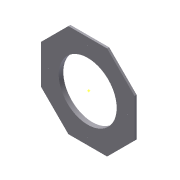
# Autodesk Inventor part: Stage3
Saved by Autodesk Inventor 2018.2 (Build 222227000, 227)
## iProperties
Created: 2018-10-31
Part Number: Stage3
Material: 3.3547 AlMg4,5Mn (AW-5083/H111)
Document SubType Name: Modeling
Designer: N.Grubert
Density: 2.66 g/cm^3
Appearance: Aluminum (gleichmäßig)
Fläche: 0 cm²
Gewicht: 0 g
Material: geeigneten Werkstoff auswählen !
Dateiname: P:\INVENTOR\Inventor 2018\Templates\ILT\Norm.ipt
Bez_eng: bolt
Bez_french: boulon
Author: N.Grubert
Autodesk Inventor part; units mm, degrees
ref_plane "YZ Plane" through (0, 0, 0) normal (1, 0, 0) x (0, 1, 0)
ref_plane "XZ Plane" through (0, 0, 0) normal (0, 1, 0) x (-1, 0, 0)
ref_plane "XY Plane" through (0, 0, 0) normal (0, 0, 1) x (1, 0, 0)
sketch "Skizze4" plane through (0, 0, 0) normal (0, 1, 0) x (-1, 0, 0)
  line L0 (-23.4031, 56.5) -> (23.4031, 56.5)
  line L1 (23.4031, 56.5) -> (56.5, 23.4031)
  line L2 (56.5, 23.4031) -> (56.5, -23.4031)
  line L3 (56.5, -23.4031) -> (23.4031, -56.5)
  line L4 (23.4031, -56.5) -> (-23.4031, -56.5)
  line L5 (-23.4031, -56.5) -> (-56.5, -23.4031)
  line L6 (-56.5, -23.4031) -> (-56.5, 23.4031)
  line L7 (-56.5, 23.4031) -> (-23.4031, 56.5)
  line L8 (0, -79.1) -> (0, 79.1) construction
  line L9 (79.1, 0) -> (-79.1, 0) construction
  circle A0 centre (0, 0) radius 35
  dimension "d4" = 113
  dimension "d5" = 70
  constraints: 16 end point, 2 coincident, 1 centre point, 18 other
  measures "d4" distance between parallel lines of L4 L0
  measures "d5" diameter of A0
extrude "Extrusion2" add sketch "Skizze4" along normal blind 2.5
sketch "Skizze5" plane through (0, 2.5, 0) normal (0, 1, 0) x (1, 0, 0)
  circle A0 centre (0, 0) radius 35 projected
  line L0 (-23.4031, -56.5) -> (23.4031, -56.5) projected
  line L1 (23.4031, -56.5) -> (56.5, -23.4031) projected
  line L2 (56.5, -23.4031) -> (56.5, 23.4031) projected
  line L3 (56.5, 23.4031) -> (23.4031, 56.5) projected
  line L4 (23.4031, 56.5) -> (-23.4031, 56.5) projected
  line L5 (-23.4031, 56.5) -> (-56.5, 23.4031) projected
  line L6 (-56.5, 23.4031) -> (-56.5, -23.4031) projected
  line L7 (-56.5, -23.4031) -> (-23.4031, -56.5) projected
  line L8 (-51.5, 21.332) -> (-21.332, 51.5)
  line L9 (-21.332, 51.5) -> (21.332, 51.5)
  line L10 (21.332, 51.5) -> (51.5, 21.332)
  line L11 (51.5, 21.332) -> (51.5, -21.332)
  line L12 (51.5, -21.332) -> (21.332, -51.5)
  line L13 (21.332, -51.5) -> (-21.332, -51.5)
  line L14 (-21.332, -51.5) -> (-51.5, -21.332)
  line L15 (-51.5, -21.332) -> (-51.5, 21.332)
  dimension "d8" = 5
  constraints: 16 end point, 7 other
  measures "d8" distance between parallel lines of L8 L5
extrude "Extrusion3" add sketch "Skizze5" along normal blind 2.5 contours L8 L9 L10 L11 L12 L13 L14 L15
sketch "Skizze6" plane through (0, 5, 0) normal (0, 1, 0) x (1, 0, 0)
  circle A0 centre (0, 0) radius 35 construction
  line L0 (-21.332, 51.5) -> (-51.5, 21.332) construction
  line L1 (-51.5, 21.332) -> (-51.5, -21.332) construction
  line L2 (-51.5, -21.332) -> (-21.332, -51.5) construction
  line L3 (-21.332, -51.5) -> (21.332, -51.5) construction
  line L4 (21.332, -51.5) -> (51.5, -21.332) construction
  line L5 (51.5, -21.332) -> (51.5, 21.332) construction
  line L6 (51.5, 21.332) -> (21.332, 51.5) construction
  line L7 (21.332, 51.5) -> (-21.332, 51.5) construction
  line L8 (0, 79.1) -> (0, -79.1) construction
  point P0 (0, 48)
  point P1 (-48, 0)
  point P2 (0, -48)
  point P3 (48, 0)
  dimension "d11" = 48
  dimension "d14" = 360
  constraints: 1 point on line, 5 other
  measures "d11" distance of point (0, 48) point (0, 0)
hole "Bohrung1" at (0, 5, -48) at (-48, 5, 0) at (0, 5, 48) at (48, 5, 0) direction (0, -1, 0) diameter 1 end through all
sketch "Skizze7" plane through (0, 2.5, 0) normal (0, 1, 0) x (1, 0, 0)
  line L0 (-21.332, 51.5) -> (21.332, 51.5) projected
  line L1 (21.332, 51.5) -> (51.5, 21.332) projected
  line L2 (51.5, 21.332) -> (51.5, -21.332) projected
  line L3 (51.5, -21.332) -> (21.332, -51.5) projected
  line L4 (21.332, -51.5) -> (-21.332, -51.5) projected
  line L5 (-21.332, -51.5) -> (-51.5, -21.332) projected
  line L6 (-51.5, -21.332) -> (-51.5, 21.332) projected
  line L7 (-51.5, 21.332) -> (-21.332, 51.5) projected
  line L8 (-23.4031, -56.5) -> (23.4031, -56.5) projected
  line L9 (23.4031, -56.5) -> (56.5, -23.4031) projected
  line L10 (56.5, -23.4031) -> (56.5, 23.4031) projected
  line L11 (56.5, 23.4031) -> (23.4031, 56.5) projected
  line L12 (23.4031, 56.5) -> (-23.4031, 56.5) projected
  line L13 (-23.4031, 56.5) -> (-56.5, 23.4031) projected
  line L14 (-56.5, 23.4031) -> (-56.5, -23.4031) projected
  line L15 (-56.5, -23.4031) -> (-23.4031, -56.5) projected
  point P0 (0, 0)
extrude "Extrusion4" cut sketch "Skizze7" against normal blind 1
sketch "Skizze8" plane through (0, 0, 0) normal (0, -1, 0) x (1, 0, 0)
  circle A0 centre (0, 48) radius 0.5 projected
  circle A1 centre (0, -48) radius 0.5 projected
  circle A2 centre (-48, 0) radius 0.5 projected
  circle A3 centre (48, 0) radius 0.5 projected
  circle A4 centre (0, 0) radius 35 projected
  line L0 (23.4031, 56.5) -> (-23.4031, 56.5) projected
  line L1 (-23.4031, 56.5) -> (-56.5, 23.4031) projected
  line L2 (-56.5, 23.4031) -> (-56.5, -23.4031) projected
  line L3 (-56.5, -23.4031) -> (-23.4031, -56.5) projected
  line L4 (-23.4031, -56.5) -> (23.4031, -56.5) projected
  line L5 (23.4031, -56.5) -> (56.5, -23.4031) projected
  line L6 (56.5, -23.4031) -> (56.5, 23.4031) projected
  line L7 (56.5, 23.4031) -> (23.4031, 56.5) projected
extrude "Extrusion5" add sketch "Skizze8" along normal blind 1
sketch "Skizze9" plane through (0, 5, 0) normal (0, 1, 0) x (1, 0, 0)
  circle A0 centre (0, -48) radius 0.5 projected
  circle A1 centre (0, 48) radius 0.5 projected
  circle A2 centre (-48, 0) radius 0.5 projected
  circle A3 centre (48, 0) radius 0.5 projected
  circle A4 centre (0, 0) radius 35 projected
  line L0 (-21.332, 51.5) -> (-51.5, 21.332) projected
  line L1 (-51.5, 21.332) -> (-51.5, -21.332) projected
  line L2 (-51.5, -21.332) -> (-21.332, -51.5) projected
  line L3 (-21.332, -51.5) -> (21.332, -51.5) projected
  line L4 (21.332, -51.5) -> (51.5, -21.332) projected
  line L5 (51.5, -21.332) -> (51.5, 21.332) projected
  line L6 (51.5, 21.332) -> (21.332, 51.5) projected
  line L7 (21.332, 51.5) -> (-21.332, 51.5) projected
extrude "Extrusion6" cut sketch "Skizze9" against normal blind 0.5 contours A0 | A1 | A2 | A3 | L7 L6 L5 L4 L3 L2 L1 L0
